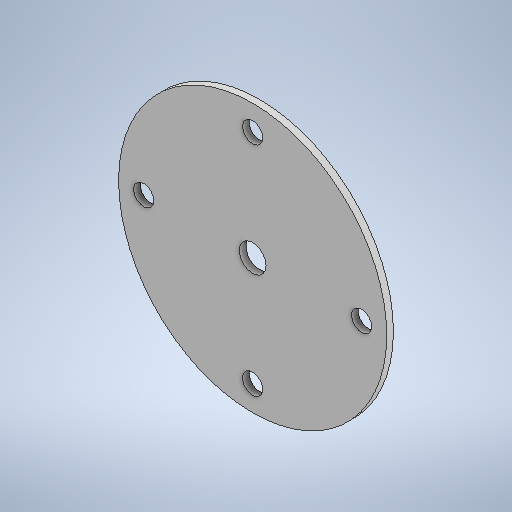
# Autodesk Inventor part: Sprocket Adapter
Saved by Autodesk Inventor 2025.2 (Build 292293000, 293)
## iProperties
Created: 2025-03-23
Part Number: Sprocket Adapter
Material: Generic
Document SubType Name: Modeling
Designer: Mathias
Density: 1 g/cm^3
Appearance: Default
Author: Mathias
Autodesk Inventor part; units mm, degrees
ref_plane "YZ Plane" through (0, 0, 0) normal (1, 0, 0) x (0, 1, 0)
ref_plane "XZ Plane" through (0, 0, 0) normal (0, 1, 0) x (-1, 0, 0)
ref_plane "XY Plane" through (0, 0, 0) normal (0, 0, 1) x (1, 0, 0)
sketch "Sketch1" plane through (0, 0, 0) normal (0, 0, 1) x (1, 0, 0)
  circle A0 centre (0, 0) radius 40
  line L0 (0, 0) -> (32.5, 0)
  line L1 (0, 0) -> (0, 32.5)
  circle A1 centre (0, 32.5) radius 3
  circle A2 centre (32.5, 0) radius 3
  circle A3 centre (0, -32.5) radius 3
  circle A4 centre (-32.5, 0) radius 3
  circle A5 centre (0, 0) radius 4
  dimension "d0" = 80
  dimension "d1" = 32.5
  dimension "d2" = 32.5
  dimension "d3" = 6
  dimension "d4" = 6
  dimension "d5" = 8
  constraints: 6 centre point, 4 coincident, 4 end point, 2 symmetric about line, 1 horizontal, 1 vertical, 2 other
  measures "d0" diameter of A0
  measures "d1" distance of L0.start L0.end
  measures "d2" distance of L0.start L1.end
  measures "d3" diameter of A1
  measures "d4" diameter of A2
  measures "d5" diameter of A5
extrude "Extrusion1" add sketch "Sketch1" along normal blind 2
body "Solid1"
